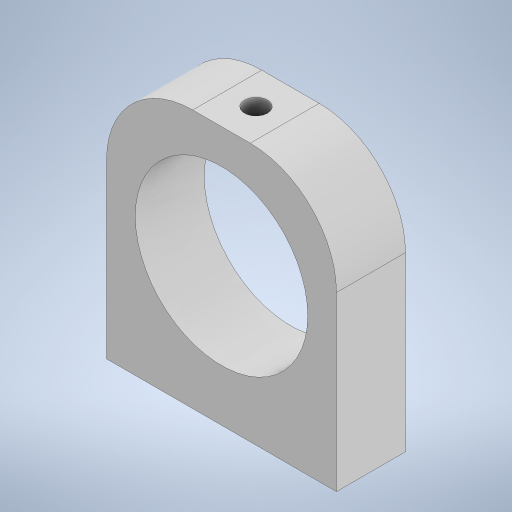
# Autodesk Inventor part: FMR_DXWD80_CPW_Halter_B
Saved by Autodesk Inventor 2023 (Build 270158000, 158)
## iProperties
Created: 2023-05-16
Part Number: FMR_DXWD80_CPW_Halter_B
Material: Generisch
Document SubType Name: Modeling
Designer: Markus Meinert
Density: 1 g/cm^3
Appearance: Vorgabe
Author: Markus Meinert
Autodesk Inventor part; units mm, degrees
ref_plane "YZ Plane" through (0, 0, 0) normal (1, 0, 0) x (0, 1, 0)
ref_plane "XZ Plane" through (0, 0, 0) normal (0, 1, 0) x (-1, 0, 0)
ref_plane "XY Plane" through (0, 0, 0) normal (0, 0, 1) x (1, 0, 0)
sketch "Skizze1" plane through (0, 0, 0) normal (0, 0, 1) x (1, 0, 0)
  line L0 (-20, -22.5) -> (20, -22.5)
  line L1 (20, -22.5) -> (20, 22.5)
  line L2 (20, 22.5) -> (-20, 22.5)
  line L3 (-20, 22.5) -> (-20, -22.5)
  line L4 (-20, -22.5) -> (20, 22.5) construction
  line L5 (20, -22.5) -> (-20, 22.5) construction
  point P0 (0, 0)
  dimension "d0" = 40
  dimension "d1" = 45
  constraints: 12 end point, 2 midpoint, 2 parallel, 1 horizontal, 1 perpendicular
  measures "d0" distance of L2.end L1.end
  measures "d1" distance of L1.end L0.end
extrude "Extrusion1" add sketch "Skizze1" along normal mid plane 12
sketch "Skizze2" plane through (0, 0, 6) normal (0, 0, 1) x (1, 0, 0)
  circle A0 centre (0, 1.5) radius 15
  line L0 (20, 22.5) -> (-20, 22.5) projected
  point P0 (0, 0)
  point P1 (0, 22.5)
  dimension "d4" = 30
  dimension "d5" = 21
  constraints: 1 centre point, 1 midpoint
  measures "d4" diameter of A0
  measures "d5" distance of A0.centre point (0, 22.5)
extrude "Extrusion2" cut sketch "Skizze2" against normal through all
sketch "Skizze3" plane through (-20, -22.5, 6) normal (0, -1, 0) x (1, 0, 0)
  line L0 (0, -12) -> (0, 0) projected
  line L1 (40, 0) -> (40, -12) projected
  point P0 (20, -6)
  point P1 (5, -6)
  point P2 (35, -6)
  dimension "d8" = 5
  dimension "d9" = 5
  constraints: 2 horizontal alignment
  measures "d8" distance from line of L0 point (5, -6)
  measures "d9" distance from line of L1 point (35, -6)
hole "Bohrung1" at (-15, -22.5, 0) at (15, -22.5, 0) direction (0, 1, 0) diameter 5.6 depth 11
sketch "Skizze4" plane through (-20, 22.5, 6) normal (0, 1, 0) x (1, 0, 0)
  point P0 (20, 6)
  point P1 (20, 6)
  constraints: 1 coincident
hole "Bohrung2" at (0, 22.5, 0) direction (0, -1, 0) diameter 4 depth 11
fillet "Rundung1" radius 15 2 edges at (-20, 22.5, 0) (20, 22.5, 0)
